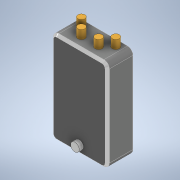
# Autodesk Inventor part: SatLab UAV_RTK
Saved by Autodesk Inventor 2022 (Build 260153000, 153)
## iProperties
Created: 2021-04-26
Part Number: SatLab UAV_RTK
Material: Generic
Document SubType Name: Modeling
Designer: lgnds
Density: 1 g/cm^3
Appearance: Default
Author: lgnds
Autodesk Inventor part; units mm, degrees
ref_plane "YZ Plane" through (0, 0, 0) normal (1, 0, 0) x (0, 1, 0)
ref_plane "XZ Plane" through (0, 0, 0) normal (0, 1, 0) x (-1, 0, 0)
ref_plane "XY Plane" through (0, 0, 0) normal (0, 0, 1) x (1, 0, 0)
sketch "Sketch1" plane through (0, 0, 0) normal (0, 0, 1) x (1, 0, 0)
  line L0 (-26, -43) -> (26, -43)
  line L1 (26, -43) -> (26, 43)
  line L2 (26, 43) -> (-26, 43)
  line L3 (-26, 43) -> (-26, -43)
  line L4 (-26, -43) -> (26, 43) construction
  line L5 (26, -43) -> (-26, 43) construction
  point P0 (0, 0)
  dimension "d0" = 52
  dimension "d1" = 86
  constraints: 12 end point, 2 midpoint, 2 parallel, 1 horizontal, 1 perpendicular
  measures "d0" distance of L1.end L2.end
  measures "d1" distance of L0.end L1.end
extrude "Extrusion1" add sketch "Sketch1" along normal blind 24
sketch "Sketch2" plane through (-26, 43, 0) normal (0, 1, 0) x (1, 0, 0)
  circle A0 centre (34, -14) radius 3.25
  circle A1 centre (42.0002, -6) radius 3.25
  line L0 (52, 0) -> (0, 0) projected
  line L1 (52, -24) -> (0, -24) projected
  line L2 (26, 4.8) -> (26, -28.8) projected
  circle A2 centre (18, -14) radius 3.25
  circle A3 centre (9.9998, -6) radius 3.25
  point P0 (26, 0)
  dimension "d4" = 6.5
  dimension "d5" = 6.5
  dimension "d6" = 6
  dimension "d7" = 10
  dimension "d8" = 8
  dimension "d9" = 16.0002
  constraints: 4 centre point, 2 symmetric about line, 2 other
  measures "d4" diameter of A0
  measures "d5" diameter of A1
  measures "d6" distance from line of L0 A1.centre
  measures "d7" distance from line of L1 A0.centre
  measures "d8" horizontal distance of point (26, 0) A0.centre
  measures "d9" horizontal distance of point (26, 0) A1.centre
extrude "Extrusion2" add sketch "Sketch2" along normal blind 8 separate body
sketch "Sketch3" plane through (0, 0, 24) normal (0, 0, 1) x (1, 0, 0)
  line L0 (0, 69.8) -> (0, -61.8) projected
  circle A0 centre (0, -35) radius 4
  line L1 (-26, -43) -> (26, -43) projected
  point P0 (0, 0)
  dimension "d12" = 8
  dimension "d13" = 8
  constraints: 1 centre point, 1 point on line
  measures "d12" diameter of A0
  measures "d13" distance from line of L1 A0.centre
extrude "Extrusion3" add sketch "Sketch3" along normal blind 4 separate body
fillet "Fillet1" radius 5 4 edges at (26, -43, 12) (-26, -43, 12) (26, 43, 12) (-26, 43, 12)
chamfer "Chamfer1" distance 2 angle 45 8 edges at (26, 0, 24) (24.5355, 41.5355, 24) (0, 43, 24) (-24.5355, 41.5355, 24) (-26, 0, 24) (-24.5355, -41.5355, 24) (0, -43, 24) (24.5355, -41.5355, 24)
equation "\"d5\" = d4"
body "Solid1"
body "Solid2"
body "Solid3"
